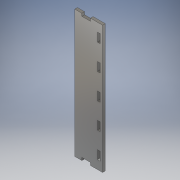
# Autodesk Inventor part: 1-8inch_Bottom1_1-Part
Saved by Autodesk Inventor 2018 (Build 220112000, 112)
## iProperties
Created: 2018-02-01
Part Number: 1-8inch_Bottom1_1-Part
Material: Generic
Document SubType Name: Modeling
Designer: Angie
Density: 1 g/cm^3
Appearance: Default
Author: Angie
Autodesk Inventor part; units mm, degrees
ref_plane "YZ Plane" through (0, 0, 0) normal (1, 0, 0) x (0, 1, 0)
ref_plane "XZ Plane" through (0, 0, 0) normal (0, 1, 0) x (-1, 0, 0)
ref_plane "XY Plane" through (0, 0, 0) normal (0, 0, 1) x (1, 0, 0)
sketch "Sketch1" plane through (0, 0, 0) normal (0, 0, 1) x (1, 0, 0)
  line L0 (-11.5, 0.5) -> (3, 0.5)
  line L1 (3, 0.5) -> (3, -148.5)
  line L2 (-11.5, -148.5) -> (-11.5, -147.1375)
  line L3 (-21.5, -147.1375) -> (-21.5, -148.5)
  line L4 (-30, -148.5) -> (-30, 0.5)
  line L5 (-30, 0.5) -> (-21.5, 0.5)
  line L6 (-21.5, 0.5) -> (-21.5, -2.5)
  line L7 (-11.5, -2.5) -> (-11.5, 0.5)
  line L8 (0, -19) -> (0, -9.66)
  line L9 (0, -49) -> (0, -39.7431)
  line L10 (0, -79) -> (0, -69.8262)
  line L11 (0, -109) -> (0, -99.9094)
  line L12 (0, -139) -> (0, -129.9925)
  line L13 (-11.5, 0.5) -> (3, 0.5)
  line L14 (3, 0.5) -> (3, -148.5)
  line L15 (-11.5, -148.5) -> (-11.5, -147.1375)
  line L16 (-21.5, -147.1375) -> (-21.5, -148.5)
  line L17 (-30, -148.5) -> (-30, 0.5)
  line L18 (-30, 0.5) -> (-21.5, 0.5)
  line L19 (-21.5, 0.5) -> (-21.5, -2.5)
  line L20 (-11.5, -2.5) -> (-11.5, 0.5)
  line L21 (0, -19) -> (0, -9.66)
  line L22 (0, -49) -> (0, -39.7431)
  line L23 (0, -79) -> (0, -69.8262)
  line L24 (0, -109) -> (0, -99.9094)
  line L25 (0, -139) -> (0, -129.9925)
  line L26 (3, 0.5) -> (3, -150.3125)
  line L27 (-30, -150.3125) -> (-30, 0.5)
  line L28 (-11.5, -150.3125) -> (-11.5, -147.1375)
  line L29 (-11.5, -147.1375) -> (-21.5, -147.1375)
  line L30 (-21.5, -147.1375) -> (-21.5, -150.3125)
  line L31 (3, -150.3125) -> (-11.5, -150.3125)
  line L32 (-21.5, -150.3125) -> (-30, -150.3125)
  line L33 (-30, 0.5) -> (-21.5, 0.5)
  line L34 (-11.5, 0.5) -> (3, 0.5)
  line L35 (-11.5, 0.5) -> (-11.5, -2.675)
  line L36 (-11.5, -2.675) -> (-21.5, -2.675)
  line L37 (-21.5, -2.675) -> (-21.5, 0.5)
  line L38 (0, 0.5) -> (-3.175, 0.5)
  line L39 (-3.175, -150.3125) -> (0, -150.3125)
  line L40 (-3.175, 0.5) -> (0, 0.5)
  line L41 (0, -9.66) -> (-3.175, -9.66)
  line L42 (0, -150.3125) -> (-3.175, -150.3125)
  line L43 (-3.175, -140.1525) -> (0, -140.1525)
  line L44 (-3.175, -140.1525) -> (0, -140.1525)
  line L45 (0, -140.1525) -> (0, -129.9925)
  line L46 (0, -129.9925) -> (-3.175, -129.9925)
  line L47 (-3.175, -129.9925) -> (-3.175, -140.1525)
  line L48 (-3.175, -9.66) -> (0, -9.66)
  line L49 (0, -9.66) -> (0, -19.82)
  line L50 (0, -19.82) -> (-3.175, -19.82)
  line L51 (-3.175, -19.82) -> (-3.175, -9.66)
  line L52 (-3.175, -19.82) -> (0, -19.82)
  line L53 (0, -39.7431) -> (-3.175, -39.7431)
  line L54 (-3.175, -39.7431) -> (0, -39.7431)
  line L55 (0, -39.7431) -> (0, -49.9031)
  line L56 (0, -49.9031) -> (-3.175, -49.9031)
  line L57 (-3.175, -49.9031) -> (-3.175, -39.7431)
  line L58 (-3.175, -49.9031) -> (0, -49.9031)
  line L59 (0, -69.8262) -> (-3.175, -69.8262)
  line L60 (-3.175, -69.8262) -> (0, -69.8262)
  line L61 (0, -69.8262) -> (0, -79.9862)
  line L62 (0, -79.9862) -> (-3.175, -79.9862)
  line L63 (-3.175, -79.9862) -> (-3.175, -69.8262)
  line L64 (-3.175, -79.9862) -> (0, -79.9862)
  line L65 (0, -99.9094) -> (-3.175, -99.9094)
  line L66 (-3.175, -99.9094) -> (0, -99.9094)
  line L67 (0, -99.9094) -> (0, -110.0694)
  line L68 (0, -110.0694) -> (-3.175, -110.0694)
  line L69 (-3.175, -110.0694) -> (-3.175, -99.9094)
  line L70 (-3.175, -110.0694) -> (0, -110.0694)
  line L71 (0, -129.9925) -> (-3.175, -129.9925)
  line L72 (-3.175, -9.66) -> (-3.175, -19.82)
  line L73 (-3.175, -39.7431) -> (-3.175, -49.9031)
  line L74 (-3.175, -69.8262) -> (-3.175, -79.9862)
  line L75 (-3.175, -99.9094) -> (-3.175, -110.0694)
  line L76 (-3.175, -129.9925) -> (-3.175, -140.1525)
  line L77 (0, -140.1525) -> (0, -129.9925)
  line L78 (0, -110.0694) -> (0, -99.9094)
  line L79 (0, -79.9862) -> (0, -69.8262)
  line L80 (0, -49.9031) -> (0, -39.7431)
  line L81 (0, -19.82) -> (0, -9.66)
  point P0 (0, 0)
  dimension "d2" = 3.175
  dimension "d4" = 10.16
  dimension "d7" = 10.16
  dimension "d9" = 10.16
  dimension "d11" = 10.16
  dimension "d12" = 19.9231
  dimension "d13" = 10.16
  constraints: 164 end point, 49 parallel, 14 horizontal, 12 perpendicular, 6 point on line
  measures "d2" distance of L0.start L35.end
  measures "d4" distance of L8.end L38.start
  measures "d7" distance of L8.end L49.end
  measures "d9" distance of L9.end L55.end
  measures "d11" distance of L10.end L61.end
  measures "d12" distance of L11.end L61.end
  measures "d13" distance of L11.end L67.end
extrude "Extrusion1" add sketch "Sketch1" along normal blind 3.175
body "Solid1"
